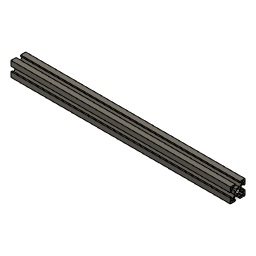
Railing (Autodesk Fusion 360 design; units mm, degrees)
Autodesk Fusion 360 part; units mm, degrees
sketch "Sketch1" plane through (0, 0, 0) normal (1, 0, 0) x (0, 0, -1)
  circle A0 centre (-17.75, 2.25) radius 1.25
  circle A1 centre (-2.25, 2.25) radius 1.25
  circle A2 centre (-17.75, 17.75) radius 1.25
  circle A3 centre (-2.25, 17.75) radius 1.25
  circle A4 centre (-10, 10) radius 2.7
  line L0 (-13.1, 0) -> (-13.1, 1.7)
  line L1 (-13.1, 1.7) -> (-15.5, 1.7)
  line L2 (-15.5, 1.7) -> (-15.5, 3.2272)
  line L3 (-13.1, 0) -> (-20, 0)
  line L4 (-13.1, 0) -> (-6.9, 0) construction
  line L5 (-10, 15.8164) -> (-10, 4.0346) construction
  line L6 (-15.4081, 10) -> (-4.6511, 10) construction
  line L7 (-16.7728, 4.5) -> (-18.3, 4.5)
  line L8 (-18.3, 4.5) -> (-18.3, 6.9)
  line L9 (-18.3, 6.9) -> (-20, 6.9)
  line L10 (-20, 6.9) -> (-20, 0)
  line L11 (0, 6.9) -> (0, 0)
  line L12 (-1.7, 6.9) -> (0, 6.9)
  line L13 (-1.7, 4.5) -> (-1.7, 6.9)
  line L14 (-3.2272, 4.5) -> (-1.7, 4.5)
  line L15 (-4.5, 1.7) -> (-4.5, 3.2272)
  line L16 (-6.9, 1.7) -> (-4.5, 1.7)
  line L17 (-6.9, 0) -> (-6.9, 1.7)
  line L18 (-6.9, 0) -> (0, 0)
  line L19 (-6.9, 20) -> (-6.9, 18.3)
  line L20 (-6.9, 18.3) -> (-4.5, 18.3)
  line L21 (-4.5, 18.3) -> (-4.5, 16.7728)
  line L22 (-3.2272, 15.5) -> (-1.7, 15.5)
  line L23 (-1.7, 15.5) -> (-1.7, 13.1)
  line L24 (-1.7, 13.1) -> (0, 13.1)
  line L25 (0, 13.1) -> (0, 20)
  line L26 (-6.9, 20) -> (0, 20)
  line L27 (-13.1, 20) -> (-13.1, 18.3)
  line L28 (-13.1, 20) -> (-20, 20)
  line L29 (-13.1, 18.3) -> (-15.5, 18.3)
  line L30 (-15.5, 18.3) -> (-15.5, 16.7728)
  line L31 (-16.7728, 15.5) -> (-18.3, 15.5)
  line L32 (-18.3, 15.5) -> (-18.3, 13.1)
  line L33 (-18.3, 13.1) -> (-20, 13.1)
  line L34 (-20, 13.1) -> (-20, 20)
  line L35 (-16.7728, 4.5) -> (-13.8, 7.4728)
  line L36 (-7.4728, 13.8) -> (-4.5, 16.7728)
  line L37 (-15.5, 16.7728) -> (-12.5272, 13.8)
  line L38 (-6.2, 7.4728) -> (-3.2272, 4.5)
  line L39 (-15.5, 3.2272) -> (-12.5272, 6.2)
  line L40 (-6.2, 12.5272) -> (-3.2272, 15.5)
  line L41 (-16.7728, 15.5) -> (-13.8, 12.5272)
  line L42 (-7.4728, 6.2) -> (-4.5, 3.2272)
  line L43 (-12.5272, 13.8) -> (-7.4728, 13.8)
  line L44 (-6.2, 12.5272) -> (-6.2, 7.4728)
  line L45 (-7.4728, 6.2) -> (-12.5272, 6.2)
  line L46 (-13.8, 7.4728) -> (-13.8, 12.5272)
  line L47 (-17.75, 17.75) -> (-2.25, 2.25) construction
  line L48 (-17.75, 2.25) -> (-2.25, 17.75) construction
  dimension "d3" = 2.5
  dimension "d13" = 15.5
  dimension "d14" = 5.4
  dimension "d16" = 2.4
  dimension "d19" = 1.7
  dimension "d21" = 3.1
  dimension "d29" = 4.5
  dimension "d30" = 1.7
  dimension "d31" = 2.4
  dimension "d32" = 4.5
  constraint equal A0 A1
  constraint equal A0 A2
  constraint equal A1 A3
  constraint perpendicular L0 L1
  constraint coincident A4.centre L5
  constraint perpendicular L5 L6
  constraint perpendicular L7 L8
  constraint symmetric L3.end L5 L11.end
  constraint symmetric L0.start L5 L4.end
  constraint symmetric L0.end L5 L16.start
  constraint symmetric L1.end L5 L15.start
  constraint symmetric L5 L7.end L13.start
  constraint symmetric L5 L8.end L12.start
  constraint symmetric L5 L9.end L11.start
  constraint symmetric L6 L11.start L24.end
  constraint symmetric L6 L11.end L25.end
  constraint symmetric L6 L12.start L23.end
  constraint symmetric L6 L13.start L22.end
  constraint symmetric L6 L15.start L20.end
  constraint symmetric L6 L16.start L19.end
  constraint symmetric L6 L4.end L19.start
  constraint symmetric L5 L19.start L27.start
  constraint symmetric L5 L19.end L27.end
  constraint symmetric L5 L20.end L29.end
  constraint symmetric L5 L22.end L31.end
  constraint symmetric L5 L23.end L32.end
  constraint symmetric L5 L24.end L33.end
  constraint symmetric L5 L25.end L28.end
  constraint collinear L35 L36
  constraint collinear L37 L38
  constraint collinear L39 L40
  constraint collinear L41 L42
  constraint horizontal L43
  constraint vertical L44
  constraint horizontal L45
  constraint vertical L46
  constraint coincident A2.centre L47.start
  constraint coincident A1.centre L47.end
  constraint coincident A0.centre L48.start
  constraint coincident A3.centre L48.end
  measures "d3" diameter of A0
  measures "d13" distance of A0.centre A1.centre
  measures "d14" diameter of A4
  measures "d16" distance of L0 L2
  measures "d19" distance of L0.start L0.end
  measures "d21" distance of L0 L5
  measures "d29" distance of L3 L7
  measures "d30" distance of L8.end L9.end
  measures "d31" distance of L7.end L8.end
  measures "d32" distance of L2 L10
extrude "Extrude1" add sketch "Sketch1" along normal blind 300
